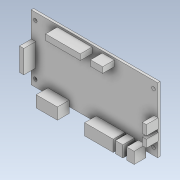
# Autodesk Inventor part: Плата контроллера
Saved by Autodesk Inventor 2021.2 (Build 252289000, 289)
## iProperties
Created: 2022-12-01
Part Number: Плата контроллера
Material: Типовые
Document SubType Name: ЛистМат
Designer: Voodoo
Mass: 20.1599 g
Surface Area: 178.763 cm^2
Volume: 20.1599 cm^3
Density: 1 g/cm^3
Sheet Metal Rule: По умолчанию_мм
Appearance: По умолчанию
Author: Voodoo
Autodesk Inventor part; units mm, degrees
ref_plane "YZ Plane" through (0, 0, 0) normal (1, 0, 0) x (0, 1, 0)
ref_plane "XZ Plane" through (0, 0, 0) normal (0, 1, 0) x (-1, 0, 0)
ref_plane "XY Plane" through (0, 0, 0) normal (0, 0, 1) x (1, 0, 0)
sketch "Эскиз1" plane through (0, 0, 0) normal (0, 0, 1) x (1, 0, 0)
  line L0 (0, 0) -> (107, 0)
  line L1 (107, 0) -> (107, 55)
  line L2 (107, 55) -> (0, 55)
  line L3 (0, 55) -> (0, 0)
  line L4 (3.5, 6) -> (103.5, 6) construction
  line L5 (103.5, 6) -> (103.5, 49) construction
  line L6 (103.5, 49) -> (3.5, 49) construction
  line L7 (3.5, 49) -> (3.5, 6) construction
  circle A0 centre (3.5, 6) radius 1.5
  circle A1 centre (3.5, 49) radius 1.5
  circle A2 centre (103.5, 49) radius 1.5
  circle A3 centre (103.5, 6) radius 1.5
  dimension "d0" = 55
  dimension "d1" = 107
  dimension "d3" = 3
  dimension "d4" = 3
  dimension "d5" = 3
  dimension "d6" = 3
  dimension "d10" = 43
  dimension "d11" = 100
  dimension "d12" = 6
  dimension "d13" = 6
  dimension "d14" = 3.5
  dimension "d16" = 3.5
  measures "d0" distance of L2.end L0.start
  measures "d1" distance of L0.start L0.end
  measures "d3" diameter of A0
  measures "d4" diameter of A1
  measures "d5" diameter of A2
  measures "d6" diameter of A3
  measures "d10" distance between parallel lines of L4 L6
  measures "d11" distance of L5.end L6.end
  measures "d12" distance between parallel lines of L0 L4
  measures "d13" distance between parallel lines of L2 L6
  measures "d14" distance between parallel lines of L3 L7
  measures "d16" distance between parallel lines of L1 L5
extrude "Пластина1" add sketch "Эскиз1" along normal blind 2
sketch "Эскиз2" plane through (0, 0, 2) normal (0, 0, 1) x (1, 0, 0)
  circle A0 centre (103.5, 6) radius 1.5 projected
  circle A1 centre (103.5, 49) radius 1.5 projected
  circle A2 centre (3.5, 49) radius 1.5 projected
  circle A3 centre (3.5, 6) radius 1.5 projected
  line L0 (0, 0) -> (0, 55) projected
  line L1 (107, 0) -> (0, 0) projected
  line L2 (107, 55) -> (107, 0) projected
  line L3 (0, 55) -> (107, 55) projected
  line L4 (97.0825, -4.8574) -> (90.7781, -4.8574)
  line L5 (90.7781, -4.8574) -> (90.7781, 4.8417)
  line L6 (90.7781, 4.8417) -> (97.0825, 4.8417)
  line L7 (97.0825, 4.8417) -> (97.0825, -4.8574)
  line L8 (87.6259, -4.8574) -> (81.3215, -4.8574)
  line L9 (81.3215, -4.8574) -> (81.3215, 4.8417)
  line L10 (81.3215, 4.8417) -> (87.6259, 4.8417)
  line L11 (87.6259, 4.8417) -> (87.6259, -4.8574)
  line L12 (79.4315, -4.8574) -> (55.1839, -4.8574)
  line L13 (55.1839, -4.8574) -> (55.1839, 4.8417)
  line L14 (55.1839, 4.8417) -> (79.4315, 4.8417)
  line L15 (79.4315, 4.8417) -> (79.4315, -4.8574)
  line L16 (32.1718, -4.8574) -> (14.1556, -4.8574)
  line L17 (14.1556, -4.8574) -> (14.1556, 4.8417)
  line L18 (14.1556, 4.8417) -> (32.1718, 4.8417)
  line L19 (32.1718, 4.8417) -> (32.1718, -4.8574)
  line L20 (51.4928, 48.572) -> (22.1532, 48.572)
  line L21 (22.1532, 48.572) -> (22.1532, 53.4215)
  line L22 (22.1532, 53.4215) -> (51.4928, 53.4215)
  line L23 (51.4928, 53.4215) -> (51.4928, 48.572)
  line L24 (70.406, 48.572) -> (60.222, 48.572)
  line L25 (60.222, 48.572) -> (60.222, 53.4215)
  line L26 (60.222, 53.4215) -> (70.406, 53.4215)
  line L27 (70.406, 53.4215) -> (70.406, 48.572)
  line L28 (107.4588, 12.3584) -> (104.0641, 12.3584)
  line L29 (104.0641, 12.3584) -> (104.0641, 18.9053)
  line L30 (104.0641, 18.9053) -> (107.4588, 18.9053)
  line L31 (107.4588, 18.9053) -> (107.4588, 12.3584)
  line L32 (107.4588, 21.3301) -> (104.0641, 21.3301)
  line L33 (104.0641, 21.3301) -> (104.0641, 29.5742)
  line L34 (104.0641, 29.5742) -> (107.4588, 29.5742)
  line L35 (107.4588, 29.5742) -> (107.4588, 21.3301)
  line L36 (3.6978, 14.141) -> (0.0607, 14.141)
  line L37 (0.0607, 14.141) -> (0.0607, 33.5391)
  line L38 (0.0607, 33.5391) -> (3.6978, 33.5391)
  line L39 (3.6978, 33.5391) -> (3.6978, 14.141)
  constraints: 72 end point, 18 parallel, 9 horizontal, 9 perpendicular, 6 point on line
extrude "Выдавливание1" add sketch "Эскиз2" along normal blind 10 separate body contours L17 L18 L19 L1 | L1 L19 L16 L17 | L34 L35 L32 L2 | L2 L32 L33 L34 | L13 L14 L15 L1 | L1 L15 L12 L13 | L30 L31 L28 L2 | L2 L28 L29 L30 | L9 L10 L11 L1 | L1 L11 L8 L9 | L5 L6 L7 L1 | L1 L7 L4 L5 | L20 L21 L22 L23 | L24 L25 L26 L27 | L36 L37 L38 L39
equation "\"d16\" = d14"
equation "\"d7\" = Толщина"
equation "\"Радиус_гибки\" = Толщина"
equation "\"Ширина_просечки\" = Толщина"
equation "\"Глубина_просечки\" = 0.5 * Толщина"
equation "\"Размер_просечки\" = 4 * Толщина"
equation "\"Мин_остаток\" = 2 * Толщина"
equation "\"Радиус_перехода\" = Радиус_гибки"
equation "\"Радиус_Якоби\" = Радиус_гибки"
equation "\"Размер_зазора\" = Толщина"
equation "\"Толщина\" = 2"
